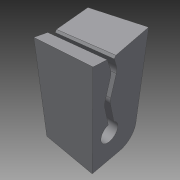
# Autodesk Inventor part: BagClip
Saved by Autodesk Inventor 2015 (Build 190159000, 159)
## iProperties
Created: 2020-03-25
Part Number: BagClip
Material: Generic
Document SubType Name: Modeling
Designer: Dominick Lee
Density: 1 g/cm^3
Appearance: Default
Author: Dominick Lee
Autodesk Inventor part; units mm, degrees
ref_plane "YZ Plane" through (0, 0, 0) normal (1, 0, 0) x (0, 1, 0)
ref_plane "XZ Plane" through (0, 0, 0) normal (0, 1, 0) x (-1, 0, 0)
ref_plane "XY Plane" through (0, 0, 0) normal (0, 0, 1) x (1, 0, 0)
sketch "Sketch1" plane through (0, 0, 0) normal (0, 1, 0) x (-1, 0, 0)
  line L0 (3, 5) -> (-3, 5)
  line L1 (-3, 5) -> (-3, -5)
  line L2 (-3, -5) -> (3, -5)
  line L3 (3, -5) -> (3, 5)
  line L4 (3, 5) -> (-3, -5) construction
  line L5 (-3, 5) -> (3, -5) construction
  point P0 (0, 0)
  dimension "d0" = 6
  dimension "d1" = 10
  constraints: 12 end point, 2 midpoint, 2 parallel, 1 horizontal, 1 perpendicular
  measures "d0" distance of L0.start L0.end
  measures "d1" distance of L1.end L0.end
extrude "Extrusion1" add sketch "Sketch1" along normal blind 5.5
sketch "Sketch2" plane through (-3, 0, -5) normal (-1, 0, 0) x (0, 0, 1)
  line L0 (0, 0) -> (0, 5.5) projected
  line L1 (0, 5.5) -> (10, 5.5) projected
  line L2 (5, 0) -> (6.2, 0)
  line L3 (0, 0) -> (10, 0) projected
  line L4 (6.2, 0) -> (7.4, 0)
  line L5 (7.4, 0) -> (8.6, 0)
  line L6 (6.4722, 1.7439) -> (8.8722, 2.3334)
  line L7 (8.8722, 2.3334) -> (9.7882, 1.9477)
  line L8 (6.4722, 1.7439) -> (6.4722, 1.1439)
  line L9 (6.4722, 1.1439) -> (4.2488, 1.7015)
  line L10 (6.4722, 1.1439) -> (8.8722, 1.7439)
  line L11 (8.8722, 1.7439) -> (10, 1.2605)
  arc A0 (4.168, 2.3613) -> (4.2488, 1.7015) centre (3.2722, 1.9167) ccw
  line L12 (6.4722, 1.7439) -> (4.168, 2.3613)
  line L13 (6.4722, 1.7439) -> (8.8578, 1.7439) construction
  line L14 (9.7882, 1.9477) -> (10, 2.0965)
  line L15 (10, 0) -> (10, 5.5) projected
  line L16 (10, 2.0965) -> (10, 1.2605)
  point P0 (10.2722, 1.9167)
  dimension "d8" = 1.2
  dimension "d9" = 1.2
  dimension "d10" = 1.2
  dimension "d17" = 0.6
  dimension "d19" = 2
  dimension "d20" = 165
  constraints: 26 end point, 5 point on line, 2 point on circle, 2 vertical, 1 centre point, 1 equal length, 1 horizontal
  measures "d8" distance of L2.start L2.end
  measures "d9" distance of L2.end L4.end
  measures "d10" distance of L4.end L5.end
  measures "d17" distance of L6.start L8.end
  measures "d19" diameter of A0
  measures "d20" angle of L13 L12
extrude "Extrusion2" cut sketch "Sketch2" against normal blind 6.5 contours L15 L11 L10 L8 L6 L7 L14 | L8 L9 A0 L12
fillet "Fillet2" radius 2 1 edges at (0, 5.5, -5)
fillet "Fillet3" radius 1 4 edges at (0, 1.7439, 3.8722) (0, 1.7439, 1.4722) (0, 1.1439, 1.4722) (0, 2.3334, 3.8722)
draft "FaceDraft2" angle 15 pull direction (0, -1, 0) faces at (-1, 3.231, 5) fixed edges at (0, 2.0965, 5)
body "Solid1"
